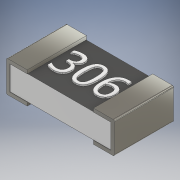
# Autodesk Inventor part: 21-1001
Saved by Autodesk Inventor 2018 (Build 220112000, 112)
## iProperties
Created: 2019-09-21
Part Number: 21-1001
Material: Copper
Document SubType Name: Modeling
Designer: Bradley
Density: 8.94 g/cm^3
Appearance: Smooth - White
Author: Bradley
Autodesk Inventor part; units mm, degrees
ref_plane "YZ Plane" through (0, 0, 0) normal (1, 0, 0) x (0, 1, 0)
ref_plane "XZ Plane" through (0, 0, 0) normal (0, 1, 0) x (-1, 0, 0)
ref_plane "XY Plane" through (0, 0, 0) normal (0, 0, 1) x (1, 0, 0)
sketch "Sketch1" plane through (0, 0, 0) normal (0, 1, 0) x (-1, 0, 0)
  line L0 (0.725, 0.175) -> (-0.725, 0.175)
  line L1 (-0.725, 0.175) -> (-0.725, -0.175)
  line L2 (-0.725, -0.175) -> (0.725, -0.175)
  line L3 (0.725, -0.175) -> (0.725, 0.175)
  line L4 (0.475, 0.175) -> (0.475, 0.225)
  line L5 (0.475, 0.225) -> (0.775, 0.225)
  line L6 (0.775, 0.225) -> (0.775, -0.225)
  line L7 (0.775, -0.225) -> (0.475, -0.225)
  line L8 (0.475, -0.225) -> (0.475, -0.175)
  line L9 (-0.475, 0.175) -> (-0.475, 0.225)
  line L10 (-0.475, 0.225) -> (-0.775, 0.225)
  line L11 (-0.775, 0.225) -> (-0.775, -0.225)
  line L12 (-0.775, -0.225) -> (-0.475, -0.225)
  line L13 (-0.475, -0.175) -> (-0.475, -0.225)
  line L14 (0.475, 0.175) -> (-0.475, 0.175)
  point P0 (0, 0)
  point P1 (0, 0.175)
  point P2 (0.725, 0)
  dimension "d0" = 1.55
  dimension "d1" = 0.05
  dimension "d2" = 0.05
  dimension "d3" = 0.45
  dimension "d4" = 0.3
  constraints: 30 end point, 12 point on line, 7 perpendicular, 3 collinear, 3 midpoint, 2 parallel, 1 horizontal, 1 horizontal alignment, 1 vertical, 1 vertical alignment
  measures "d0" distance between parallel lines of L11 L6
  measures "d1" distance of L7.end L8.end
  measures "d2" distance between parallel lines of L6 L3
  measures "d3" distance of L5.end L6.end
  measures "d4" distance of L6.end L7.end
extrude "Extrusion1" add sketch "Sketch1" along normal mid plane 0.85 contours L0 L4 L5 L6 L7 L8 L2 L3 | L0 L1 L2 L13 L12 L11 L10 L9
extrude "Extrusion2" add sketch "Sketch1" along normal mid plane 0.84 contours L3 L2 L1 L0
sketch "Sketch2" plane through (-0.475, -0.42, 0.175) normal (0, 0, 1) x (1, 0, 0)
  line L0 (0, 0) -> (0, 0.84) projected
  line L1 (0.95, 0) -> (0, 0) projected
  line L2 (0.95, 0) -> (0.95, 0.84) projected
  line L3 (0, 0.84) -> (0.95, 0.84) projected
  line L4 (0, 0.42) -> (0.95, 0.42) construction
  spline S0 degree 2 poles (0.1619, 0.5821) (0.1473, 0.5821) (0.1184, 0.5749) (0.1045, 0.5694) knots 0 0 0 1 2 2 2
  spline S1 degree 2 poles (0.1045, 0.5694) (0.0915, 0.5639) (0.0724, 0.5523) (0.065, 0.5471) knots 0 0 0 1 2 2 2
  line L5 (0.065, 0.5471) -> (0.0617, 0.5471)
  line L6 (0.0617, 0.5471) -> (0.0617, 0.6038)
  spline S2 degree 2 poles (0.0617, 0.6038) (0.0792, 0.6132) (0.1392, 0.6284) (0.1661, 0.6284) knots 0 0 0 1 2 2 2
  spline S3 degree 2 poles (0.1661, 0.6284) (0.1933, 0.6284) (0.2338, 0.6174) (0.2504, 0.6057) knots 0 0 0 1 2 2 2
  spline S4 degree 2 poles (0.2504, 0.6057) (0.2679, 0.5931) (0.286, 0.5565) (0.286, 0.5318) knots 0 0 0 1 2 2 2
  spline S5 degree 2 poles (0.286, 0.5318) (0.286, 0.4988) (0.2426, 0.4488) (0.2121, 0.4424) knots 0 0 0 1 2 2 2
  line L7 (0.2121, 0.4424) -> (0.2121, 0.4385)
  spline S6 degree 2 poles (0.2121, 0.4385) (0.2248, 0.4359) (0.2536, 0.4242) (0.2659, 0.4125) knots 0 0 0 1 2 2 2
  spline S7 degree 2 poles (0.2659, 0.4125) (0.2782, 0.4012) (0.2938, 0.3649) (0.2938, 0.3386) knots 0 0 0 1 2 2 2
  spline S8 degree 2 poles (0.2938, 0.3386) (0.2938, 0.3117) (0.2753, 0.266) (0.2585, 0.2485) knots 0 0 0 1 2 2 2
  spline S9 degree 2 poles (0.2585, 0.2485) (0.241, 0.2304) (0.1914, 0.2116) (0.1599, 0.2116) knots 0 0 0 1 2 2 2
  spline S10 degree 2 poles (0.1599, 0.2116) (0.1298, 0.2116) (0.0708, 0.2262) (0.0507, 0.2362) knots 0 0 0 1 2 2 2
  line L8 (0.0507, 0.2362) -> (0.0507, 0.2929)
  line L9 (0.0507, 0.2929) -> (0.0546, 0.2929)
  spline S11 degree 2 poles (0.0546, 0.2929) (0.0714, 0.2806) (0.1285, 0.2579) (0.1567, 0.2579) knots 0 0 0 1 2 2 2
  spline S12 degree 2 poles (0.1567, 0.2579) (0.1732, 0.2579) (0.2063, 0.2683) (0.2173, 0.2803) knots 0 0 0 1 2 2 2
  spline S13 degree 2 poles (0.2173, 0.2803) (0.228, 0.2923) (0.2393, 0.3208) (0.2393, 0.3425) knots 0 0 0 1 2 2 2
  spline S14 degree 2 poles (0.2393, 0.3425) (0.2393, 0.3642) (0.2267, 0.3924) (0.2154, 0.4006) knots 0 0 0 1 2 2 2
  spline S15 degree 2 poles (0.2154, 0.4006) (0.204, 0.4087) (0.1732, 0.4148) (0.1551, 0.4148) knots 0 0 0 1 2 2 2
  line L10 (0.1551, 0.4148) -> (0.1324, 0.4148)
  line L11 (0.1324, 0.4148) -> (0.1324, 0.4592)
  line L12 (0.1324, 0.4592) -> (0.1502, 0.4592)
  spline S16 degree 2 poles (0.1502, 0.4592) (0.1862, 0.4592) (0.2316, 0.4936) (0.2316, 0.5263) knots 0 0 0 1 2 2 2
  spline S17 degree 2 poles (0.2316, 0.5263) (0.2316, 0.5416) (0.2199, 0.5633) (0.2105, 0.5698) knots 0 0 0 1 2 2 2
  spline S18 degree 2 poles (0.2105, 0.5698) (0.2004, 0.5766) (0.1758, 0.5821) (0.1619, 0.5821) knots 0 0 0 1 2 2 2
  spline S19 degree 2 poles (0.603, 0.42) (0.603, 0.3124) (0.5405, 0.2116) (0.4753, 0.2116) knots 0 0 0 1 2 2 2
  spline S20 degree 2 poles (0.4753, 0.2116) (0.4092, 0.2116) (0.3473, 0.3143) (0.3473, 0.4197) knots 0 0 0 1 2 2 2
  spline S21 degree 2 poles (0.3473, 0.4197) (0.3473, 0.5279) (0.4098, 0.6281) (0.4753, 0.6281) knots 0 0 0 1 2 2 2
  spline S22 degree 2 poles (0.4753, 0.6281) (0.5411, 0.6281) (0.603, 0.5244) (0.603, 0.42) knots 0 0 0 1 2 2 2
  spline S23 degree 2 poles (0.5343, 0.2981) (0.5421, 0.3179) (0.5486, 0.3788) (0.5486, 0.42) knots 0 0 0 1 2 2 2
  spline S24 degree 2 poles (0.5486, 0.42) (0.5486, 0.4612) (0.5421, 0.5218) (0.534, 0.5422) knots 0 0 0 1 2 2 2
  spline S25 degree 2 poles (0.534, 0.5422) (0.5259, 0.5626) (0.4977, 0.5837) (0.4753, 0.5837) knots 0 0 0 1 2 2 2
  spline S26 degree 2 poles (0.4753, 0.5837) (0.453, 0.5837) (0.4241, 0.5626) (0.4157, 0.5416) knots 0 0 0 1 2 2 2
  spline S27 degree 2 poles (0.4157, 0.5416) (0.4076, 0.5211) (0.4017, 0.4589) (0.4017, 0.4197) knots 0 0 0 1 2 2 2
  spline S28 degree 2 poles (0.4017, 0.4197) (0.4017, 0.3775) (0.4069, 0.3211) (0.4154, 0.2991) knots 0 0 0 1 2 2 2
  spline S29 degree 2 poles (0.4154, 0.2991) (0.4231, 0.2783) (0.452, 0.256) (0.4753, 0.256) knots 0 0 0 1 2 2 2
  spline S30 degree 2 poles (0.4753, 0.256) (0.4974, 0.256) (0.5262, 0.2771) (0.5343, 0.2981) knots 0 0 0 1 2 2 2
  spline S31 degree 2 poles (0.9071, 0.3497) (0.9071, 0.3189) (0.8867, 0.2667) (0.8695, 0.2492) knots 0 0 0 1 2 2 2
  spline S32 degree 2 poles (0.8695, 0.2492) (0.8517, 0.2307) (0.8069, 0.2116) (0.78, 0.2116) knots 0 0 0 1 2 2 2
  spline S33 degree 2 poles (0.78, 0.2116) (0.7531, 0.2116) (0.7087, 0.2297) (0.6919, 0.2479) knots 0 0 0 1 2 2 2
  spline S34 degree 2 poles (0.6919, 0.2479) (0.6711, 0.2696) (0.6478, 0.3425) (0.6478, 0.3957) knots 0 0 0 1 2 2 2
  spline S35 degree 2 poles (0.6478, 0.3957) (0.6478, 0.4479) (0.6692, 0.5318) (0.6915, 0.5629) knots 0 0 0 1 2 2 2
  spline S36 degree 2 poles (0.6915, 0.5629) (0.7132, 0.5934) (0.782, 0.6275) (0.827, 0.6275) knots 0 0 0 1 2 2 2
  spline S37 degree 2 poles (0.827, 0.6275) (0.8403, 0.6275) (0.8637, 0.6249) (0.8724, 0.6219) knots 0 0 0 1 2 2 2
  line L13 (0.8724, 0.6219) -> (0.8724, 0.5704)
  line L14 (0.8724, 0.5704) -> (0.8701, 0.5704)
  spline S38 degree 2 poles (0.8701, 0.5704) (0.8627, 0.5743) (0.8355, 0.5811) (0.8199, 0.5811) knots 0 0 0 1 2 2 2
  spline S39 degree 2 poles (0.8199, 0.5811) (0.77, 0.5811) (0.7087, 0.5137) (0.7029, 0.4476) knots 0 0 0 1 2 2 2
  spline S40 degree 2 poles (0.7029, 0.4476) (0.722, 0.4608) (0.7622, 0.4754) (0.7862, 0.4754) knots 0 0 0 1 2 2 2
  spline S41 degree 2 poles (0.7862, 0.4754) (0.8095, 0.4754) (0.8445, 0.466) (0.8637, 0.4518) knots 0 0 0 1 2 2 2
  spline S42 degree 2 poles (0.8637, 0.4518) (0.8857, 0.4352) (0.9071, 0.384) (0.9071, 0.3497) knots 0 0 0 1 2 2 2
  spline S43 degree 2 poles (0.8526, 0.3474) (0.8526, 0.372) (0.8397, 0.4054) (0.8254, 0.4171) knots 0 0 0 1 2 2 2
  spline S44 degree 2 poles (0.8254, 0.4171) (0.8147, 0.4255) (0.7881, 0.431) (0.7742, 0.431) knots 0 0 0 1 2 2 2
  spline S45 degree 2 poles (0.7742, 0.431) (0.7554, 0.431) (0.7201, 0.4197) (0.7029, 0.409) knots 0 0 0 1 2 2 2
  spline S46 degree 2 poles (0.7029, 0.409) (0.7026, 0.4031) (0.7019, 0.3921) (0.7019, 0.3837) knots 0 0 0 1 2 2 2
  spline S47 degree 2 poles (0.7019, 0.3837) (0.7019, 0.3422) (0.7181, 0.2913) (0.7304, 0.278) knots 0 0 0 1 2 2 2
  spline S48 degree 2 poles (0.7304, 0.278) (0.7418, 0.2654) (0.7664, 0.2553) (0.7803, 0.2553) knots 0 0 0 1 2 2 2
  spline S49 degree 2 poles (0.7803, 0.2553) (0.8128, 0.2553) (0.8526, 0.3014) (0.8526, 0.3474) knots 0 0 0 1 2 2 2
  point P0 (0.475, 0.42)
  constraints: 2 end point, 2 midpoint, 1 horizontal
extrude "Extrusion3" add sketch "Sketch2" along normal blind 0.02 contours S0 S1 L5 L6 S2 S3 S4 S5 L7 S6 S7 S8 S9 S10 L8 L9 S11 S12 S13 S14 S15 L10 L11 L12 S16 S17 S18 | S19 S20 S21 S22 | S31 S32 S33 S34 S35 S36 S37 L13 L14 S38 S39 S40 S41 S42
fillet "Fillet1" radius 0.02 4 edges at (-0.775, 0, 0.225) (-0.775, 0, -0.225) (0.775, 0, 0.225) (0.775, 0, -0.225)
equation "\"d2\" = d1"
body "Solid1"
